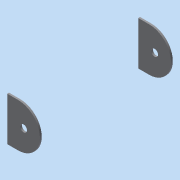
# Autodesk Inventor part: Side Beam
Saved by Autodesk Inventor 2015 (Build 190159000, 159)
## iProperties
Created: 2014-09-21
Part Number: Side Beam
Material: Generic
Document SubType Name: Modeling
Designer: Kris
Density: 1 g/cm^3
Appearance: Default
Author: Kris
Autodesk Inventor part; units mm, degrees
ref_plane "YZ Plane" through (0, 0, 0) normal (1, 0, 0) x (0, 1, 0)
ref_plane "XZ Plane" through (0, 0, 0) normal (0, 1, 0) x (-1, 0, 0)
sketch "Side Element" plane through (0, 0, 0) normal (0, 0, 1) x (1, 0, 0)
  line L0 (0, 0) -> (38.1, 0)
  line L1 (38.1, 0) -> (38.1, 50.8)
  line L2 (38.1, 50.8) -> (0, 50.8)
  line L3 (0, 50.8) -> (0, 0)
  dimension "d0" = 38.1
  dimension "d1" = 50.8
  constraints: 8 end point, 2 parallel, 1 horizontal, 1 perpendicular
  measures "d0" distance of L2.end L1.end
  measures "d1" distance of L0.end L1.end
extrude "Extrusion1" add sketch "Side Element" against normal blind 2.1082
fillet "Fillet1" radius 25.4 1 edges at (38.1, 50.8, -1.0541)
ref_plane "Work Plane2" through (0, 0, -152.4) normal (0, 0, 1) x (1, 0, 0)
sketch "Sketch6" plane through (0, 0, -152.4) normal (0, 0, 1) x (1, 0, 0)
  line L0 (0, 0) -> (38.1293, 0)
  line L1 (38.1293, 0) -> (38.1293, 50.8)
  line L2 (38.1293, 50.8) -> (0, 50.8)
  line L3 (0, 50.8) -> (0, 0)
  dimension "d23" = 50.8
  constraints: 8 end point, 2 parallel, 1 horizontal, 1 perpendicular
  measures "d23" distance of L0.end L1.end
extrude "Extrusion5" add sketch "Sketch6" against normal blind 2.1082
fillet "Fillet3" radius 25.4 1 edges at (38.1293, 50.8, -153.4541)
sketch "Sketch7" plane through (0, 0, -152.4) normal (0, 0, 1) x (1, 0, 0)
  circle A0 centre (19.0793, 25.4) radius 4
  line L0 (0, 0) -> (38.1293, 0) projected
  line L1 (38.1293, 0) -> (38.1293, 25.4) projected
  dimension "d27" = 8
  dimension "d28" = 25.4
  dimension "d29" = 19.05
  constraints: 1 centre point
  measures "d27" diameter of A0
  measures "d28" distance from line of A0.centre L0
  measures "d29" distance from line of L1 A0.centre
extrude "Extrusion6" cut sketch "Sketch7" against normal blind 2.1082
sketch "Sketch8" plane through (0, 0, -2.1082) normal (0, 0, -1) x (-1, 0, 0)
  circle A0 centre (-19.05, 25.4) radius 4
  line L0 (-38.1, 0) -> (0, 0) projected
  line L1 (0, 0) -> (0, 50.8) projected
  dimension "d32" = 8
  dimension "d33" = 25.4
  dimension "d34" = 19.05
  constraints: 1 centre point
  measures "d32" diameter of A0
  measures "d33" distance from line of A0.centre L0
  measures "d34" distance from line of A0.centre L1
extrude "Extrusion7" cut sketch "Sketch8" against normal blind 2.1082
fillet "Fillet4" radius 25.4 1 edges at (38.1, 0, -1.0541)
fillet "Fillet5" radius 25.4 1 edges at (38.1293, 0, -153.4541)
body "Solid1"
